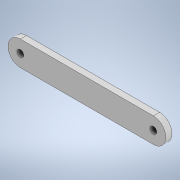
# Autodesk Inventor part: Eslabon
Saved by Autodesk Inventor 2021 (Build 250183000, 183)
## iProperties
Created: 2022-01-12
Part Number: Eslabon
Material: Generic
Document SubType Name: Modeling
Designer: Yeison
Density: 1 g/cm^3
Appearance: Default
Author: Yeison
Autodesk Inventor part; units mm, degrees
ref_plane "YZ Plane" through (0, 0, 0) normal (1, 0, 0) x (0, 1, 0)
ref_plane "XZ Plane" through (0, 0, 0) normal (0, 1, 0) x (-1, 0, 0)
ref_plane "XY Plane" through (0, 0, 0) normal (0, 0, 1) x (1, 0, 0)
sketch "Sketch1" plane through (0, 0, 0) normal (0, 0, 1) x (1, 0, 0)
  line L0 (107.5, -20) -> (-107.5, -20)
  line L1 (-107.5, -20) -> (-107.5, 20)
  line L2 (-107.5, 20) -> (107.5, 20)
  line L3 (107.5, 20) -> (107.5, -20)
  line L4 (107.5, -20) -> (-107.5, 20) construction
  line L5 (-107.5, -20) -> (107.5, 20) construction
  arc A0 (-107.5, 20) -> (-107.5, -20) centre (-107.5, 0) ccw
  arc A1 (107.5, -20) -> (107.5, 20) centre (107.5, 0) ccw
  circle A2 centre (-107.5, 0) radius 5.5
  circle A3 centre (107.5, 0) radius 5.5
  point P0 (0, 0)
  dimension "d0" = 215
  dimension "d1" = 40
  dimension "d4" = 11
  dimension "d5" = 11
  constraints: 12 end point, 4 centre point, 4 point on circle, 2 coincident, 2 midpoint, 2 parallel, 1 horizontal, 1 perpendicular
  measures "d0" distance of L1.end L2.end
  measures "d1" distance of L0.end L1.end
  measures "d4" diameter of A2
  measures "d5" diameter of A3
extrude "Extrusion1" add sketch "Sketch1" along normal blind 10 contours L0 L1 A2 L2 L3 A3 | L3 A3 A1 | A0 L1 A2
body "Solid1"
